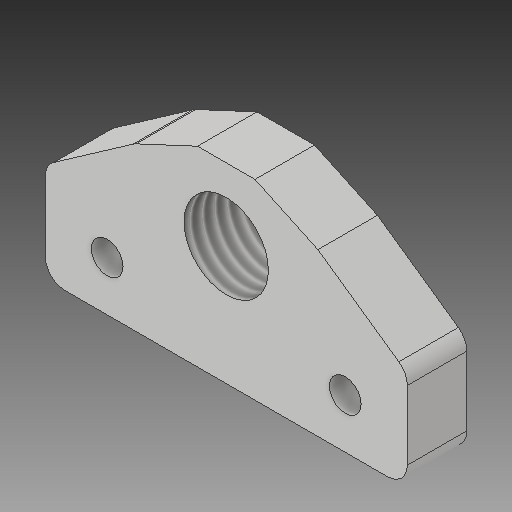
# Autodesk Inventor part: pshfit-mount-acrylic
Saved by Autodesk Inventor 2018 (Build 220112000, 112)
## iProperties
Created: 2016-07-07
Part Number: pshfit-mount-acrylic
Material: Generic
Document SubType Name: Modeling
Designer: joshmamo
Density: 1 g/cm^3
Appearance: Default
Mass: 2.99682 g
Surface Area: 18.5729 cm^2
Volume: 2.99682 cm^3
Author: joshmamo
Autodesk Inventor part; units mm, degrees
ref_plane "YZ Plane" through (0, 0, 0) normal (1, 0, 0) x (0, 1, 0)
ref_plane "XZ Plane" through (0, 0, 0) normal (0, 1, 0) x (-1, 0, 0)
ref_plane "XY Plane" through (0, 0, 0) normal (0, 0, 1) x (1, 0, 0)
sketch "Sketch1" plane through (0, 0, 0) normal (0, 0, 1) x (1, 0, 0)
  line L0 (37.7292, 11.7639) -> (29.5714, 17.4761)
  line L1 (29.5714, 17.4761) -> (23.2272, 20.4344)
  line L2 (23.2272, 20.4344) -> (17.4366, 20.4344)
  line L3 (17.4366, 20.4344) -> (11.251, 17.55)
  arc A0 (11.251, 17.55) -> (10.9491, 17.3757) centre (12.0963, 15.7374) ccw
  line L4 (10.9491, 17.3757) -> (2.9346, 11.7639)
  arc A1 (2.9346, 11.7639) -> (2.0818, 10.1256) centre (4.0818, 10.1256) ccw
  line L5 (2.0818, 10.1256) -> (2.0818, 3.1667)
  arc A2 (2.0818, 3.1667) -> (4.0818, 1.1667) centre (4.0818, 3.1667) ccw
  line L6 (4.0818, 1.1667) -> (36.5821, 1.1667)
  arc A3 (36.5821, 1.1667) -> (38.5821, 3.1667) centre (36.5821, 3.1667) ccw
  line L7 (38.5821, 3.1667) -> (38.5821, 10.1256)
  arc A4 (38.5821, 10.1256) -> (37.7292, 11.7639) centre (36.5821, 10.1256) ccw
  circle A5 centre (8.3339, 6.1667) radius 1.6
  circle A6 centre (32.3301, 6.1667) radius 1.6
  circle A7 centre (20.3315, 13.1667) radius 4.25
  point P0 (0, 0)
  constraints: 16 end point, 10 point on circle, 8 centre point
extrude "Extrusion1" add sketch "Sketch1" along normal blind 6
thread "Thread1" size "M9x1.25" class "6H" standard "ANSI Metric M Profile" full length
body "Solid1"
